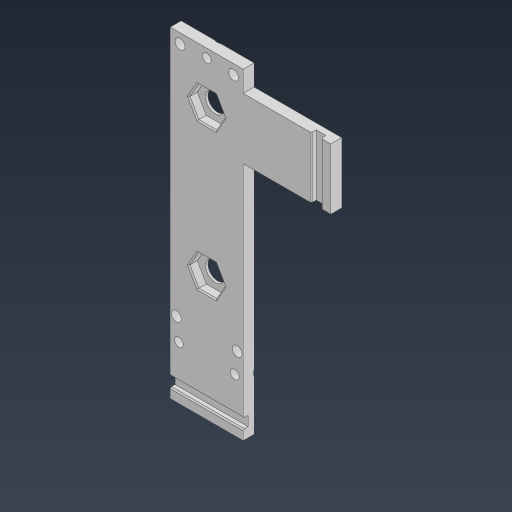
# Autodesk Inventor part: fusion_hold
Saved by Autodesk Inventor 2023 (Build 270158000, 158)
## iProperties
Created: 2025-12-26
Part Number: fusion_hold
Material: Generic
Document SubType Name: Modeling
Designer: szymo
Density: 1 g/cm^3
Appearance: Default
Author: szymo
Autodesk Inventor part; units mm, degrees
ref_plane "YZ Plane" through (0, 0, 0) normal (1, 0, 0) x (0, 1, 0)
ref_plane "XZ Plane" through (0, 0, 0) normal (0, 1, 0) x (-1, 0, 0)
ref_plane "XY Plane" through (0, 0, 0) normal (0, 0, 1) x (1, 0, 0)
ref_plane "Work Plane1" through (0, 0, 0) normal (0, 0, 1) x (1, 0, 0)
sketch "Sketch1" plane through (0, 0, 0) normal (0, 0, 1) x (1, 0, 0)
  line L0 (-10, -38.8003) -> (-10, -16.5003) projected
  arc A0 (-10, -38.8003) -> (-7.75, -41.0997) centre (-7.7, -38.8003) ccw projected
  arc A1 (-7.75, -41.0997) -> (-5.5, -38.8003) centre (-7.8, -38.8003) ccw projected
  line L1 (-5.5, -30.0003) -> (-5.5, -38.8003) projected
  arc A2 (5.5, -30.0003) -> (-5.5, -30.0003) centre (0, -30.0003) ccw projected
  line L2 (5.5, -38.8003) -> (5.5, -30.0003) projected
  arc A3 (5.5, -38.8003) -> (7.75, -41.0997) centre (7.8, -38.8003) ccw projected
  arc A4 (7.75, -41.0997) -> (10, -38.8003) centre (7.7, -38.8003) ccw projected
  line L3 (10, -16.5003) -> (10, -38.8003) projected
  line L4 (3.75, -16.5003) -> (10, -16.5003) projected
  line L5 (3.75, -12.5003) -> (3.75, -16.5003) projected
  line L6 (7.5, -12.5003) -> (3.75, -12.5003) projected
  line L7 (7.5, -10.0003) -> (7.5, -12.5003) projected
  line L8 (1.75, -10.0003) -> (7.5, -10.0003) projected
  arc A5 (1.25, -9.5003) -> (1.75, -10.0003) centre (1.75, -9.5003) ccw projected
  line L9 (1.25, 9.4997) -> (1.25, -9.5003) projected
  arc A6 (1.75, 9.9997) -> (1.25, 9.4997) centre (1.75, 9.4997) ccw projected
  line L10 (7.5, 9.9997) -> (1.75, 9.9997) projected
  line L11 (7.5, 12.4997) -> (7.5, 9.9997) projected
  line L12 (3.75, 12.4997) -> (7.5, 12.4997) projected
  line L13 (3.75, 16.4997) -> (3.75, 12.4997) projected
  line L14 (10, 16.4997) -> (3.75, 16.4997) projected
  line L15 (10, 21.6997) -> (10, 16.4997) projected
  arc A7 (10, 21.6997) -> (7.2, 24.4997) centre (7.2, 21.6997) ccw projected
  line L16 (0, 24.4997) -> (7.2, 24.4997) projected
  arc A8 (0, 35.4997) -> (0, 24.4997) centre (0, 29.9997) ccw projected
  line L17 (7.2, 35.4997) -> (0, 35.4997) projected
  arc A9 (7.2, 35.4997) -> (7.2, 41.0997) centre (7.2, 38.2997) ccw projected
  line L18 (-10, 41.0997) -> (7.2, 41.0997) projected
  line L19 (-10, 16.4997) -> (-10, 41.0997) projected
  line L20 (-3.75, 16.4997) -> (-10, 16.4997) projected
  line L21 (-3.75, 12.4997) -> (-3.75, 16.4997) projected
  line L22 (-7.5, 12.4997) -> (-3.75, 12.4997) projected
  line L23 (-7.5, 9.9997) -> (-7.5, 12.4997) projected
  line L24 (-1.75, 9.9997) -> (-7.5, 9.9997) projected
  arc A10 (-1.25, 9.4997) -> (-1.75, 9.9997) centre (-1.75, 9.4997) ccw projected
  line L25 (-1.25, -9.5003) -> (-1.25, 9.4997) projected
  arc A11 (-1.75, -10.0003) -> (-1.25, -9.5003) centre (-1.75, -9.5003) ccw projected
  line L26 (-7.5, -10.0003) -> (-1.75, -10.0003) projected
  line L27 (-7.5, -12.5003) -> (-7.5, -10.0003) projected
  line L28 (-3.75, -12.5003) -> (-7.5, -12.5003) projected
  line L29 (-3.75, -16.5003) -> (-3.75, -12.5003) projected
  line L30 (-10, -16.5003) -> (-3.75, -16.5003) projected
  line L31 (15, 51.0997) -> (-15, 51.0997)
  line L32 (-15, 51.0997) -> (-15, -81.0997)
  line L33 (-15, -81.0997) -> (15, -81.0997)
  line L34 (15, -81.0997) -> (15, 51.0997)
  circle A12 centre (0, 29.9997) radius 4
  circle A13 centre (0, -30.0003) radius 4
  line L35 (15, 18.4997) -> (-15, 18.4997)
  line L36 (-15, -18.5003) -> (15, -18.5003)
  line L37 (13.1, 18.4997) -> (13.1, -18.5003)
  line L38 (-13.1, -18.5003) -> (-13.1, 18.4997)
  line L39 (11.1, 15.3997) -> (11.1, -15.4003) projected
  line L40 (-11.1, 15.3997) -> (-11.1, -15.4003) projected
  point P0 (0, 0)
  point P1 (10, -18.5003)
  point P2 (-10, -18.5003)
  point P3 (-10, 18.4997)
  point P4 (10, 18.4997)
  dimension "d5" = 8
  dimension "d6" = 8
  dimension "d8" = 5
  dimension "d9" = 10
  dimension "d10" = 5
  dimension "d11" = 40
  dimension "d12" = 2
  dimension "d13" = 2
  dimension "d14" = 2
  dimension "d15" = 2
  constraints: 16 end point, 8 point on line, 5 parallel, 5 perpendicular, 2 centre point, 2 coincident, 1 horizontal
  measures "d5" diameter of A12
  measures "d6" diameter of A13
  measures "d8" distance between parallel lines of L19 L32
  measures "d9" distance between parallel lines of L31 L18
  measures "d10" distance between parallel lines of L34 L15
  measures "d11" distance from line of L33 A0.end
  measures "d12" distance between parallel lines of L20 L35
  measures "d13" distance between parallel lines of L36 L4
  measures "d14" distance between parallel lines of L39 L37
  measures "d15" distance between parallel lines of L40 L38
extrude "Extrusion1" add sketch "Sketch1" along normal blind 1 contours A0 A1 L1 A2 L2 A3 A4 L3 L36 L34 L33 L32 L0 | L0 L36 L3 A4 A3 L2 A2 L1 A1 A0 | L36 L32 L35 L38 | L35 L32 L31 L34 L15 A7 L16 A8 L17 A9 L18 L19 | L37 L35 L34 L36 | L19 L18 A9 L17 A8 L16 A7 L15 L35
sketch "Sketch2" plane through (0, 0, 1) normal (0, 0, 1) x (1, 0, 0)
  line L0 (15, 51.0997) -> (-15, 51.0997) projected
  line L1 (-15, 51.0997) -> (-15, -81.0997) projected
  line L2 (-15, -81.0997) -> (15, -81.0997) projected
  line L3 (15, -81.0997) -> (15, 51.0997) projected
  circle A0 centre (0, -30.0003) radius 4 projected
  line L4 (13.1, -18.5003) -> (-13.1, -18.5003) projected
  line L5 (-13.1, -18.5003) -> (-13.1, 18.4997) projected
  line L6 (-13.1, 18.4997) -> (13.1, 18.4997) projected
  line L7 (13.1, 18.4997) -> (13.1, -18.5003) projected
  circle A1 centre (0, 29.9997) radius 4 projected
  line L8 (3.695, 36.3997) -> (7.3901, 29.9997)
  line L9 (7.3901, 29.9997) -> (3.695, 23.5997)
  line L10 (3.695, 23.5997) -> (-3.695, 23.5997)
  line L11 (-3.695, 23.5997) -> (-7.3901, 29.9997)
  line L12 (-7.3901, 29.9997) -> (-3.695, 36.3997)
  line L13 (-3.695, 36.3997) -> (3.695, 36.3997)
  line L14 (7.3901, -30.0003) -> (3.695, -36.4003)
  line L15 (3.695, -36.4003) -> (-3.695, -36.4003)
  line L16 (-3.695, -36.4003) -> (-7.3901, -30.0003)
  line L17 (-7.3901, -30.0003) -> (-3.695, -23.6003)
  line L18 (-3.695, -23.6003) -> (3.695, -23.6003)
  line L19 (3.695, -23.6003) -> (7.3901, -30.0003)
  point P0 (0, 0)
  point P1 (0, 29.9997)
  point P2 (0, -30.0003)
  dimension "d20" = 0
  dimension "d21" = 0
  dimension "d22" = 12.8
  dimension "d23" = 12.8
  constraints: 24 end point, 2 coincident, 26 other
  measures "d20" angle of L2 L15
  measures "d21" angle of L0 L13
  measures "d22" distance between parallel lines of L10 L13
  measures "d23" distance between parallel lines of L15 L18
extrude "Extrusion2" add sketch "Sketch2" along normal blind 2 contours L3 L2 L1 L0
sketch "Sketch6" plane through (0, 0, 3) normal (0, 0, 1) x (1, 0, 0)
  line L0 (-15, 51.0997) -> (-15, -81.0997) projected
  line L1 (-15, -81.0997) -> (15, -81.0997) projected
  line L2 (15, -81.0997) -> (15, 51.0997) projected
  line L3 (15, 51.0997) -> (-15, 51.0997) projected
  line L4 (7.3901, -30.0003) -> (3.695, -36.4003) projected
  line L5 (3.695, -36.4003) -> (-3.695, -36.4003) projected
  line L6 (-3.695, -36.4003) -> (-7.3901, -30.0003) projected
  line L7 (-7.3901, -30.0003) -> (-3.695, -23.6003) projected
  line L8 (-3.695, -23.6003) -> (3.695, -23.6003) projected
  line L9 (3.695, -23.6003) -> (7.3901, -30.0003) projected
  line L10 (3.695, 36.3997) -> (7.3901, 29.9997) projected
  line L11 (7.3901, 29.9997) -> (3.695, 23.5997) projected
  line L12 (3.695, 23.5997) -> (-3.695, 23.5997) projected
  line L13 (-3.695, 23.5997) -> (-7.3901, 29.9997) projected
  line L14 (-7.3901, 29.9997) -> (-3.695, 36.3997) projected
  line L15 (-3.695, 36.3997) -> (3.695, 36.3997) projected
  line L16 (13.1, -18.5003) -> (-13.1, -18.5003) projected
  line L17 (-13.1, -18.5003) -> (-13.1, 18.4997) projected
  line L18 (-13.1, 18.4997) -> (13.1, 18.4997) projected
  line L19 (13.1, 18.4997) -> (13.1, -18.5003) projected
  point P0 (0, 0)
extrude "Extrusion3" add sketch "Sketch6" along normal blind 1.5 contours L3 L2 L1 L0 | L16 L17 L18 L19
sketch "Sketch7" plane through (0, 0, 0) normal (0, 0, -1) x (-1, 0, 0)
  line L0 (15, -81.0997) -> (-15, -81.0997) projected
  line L1 (0, -81.0997) -> (0, 51.0997)
  line L2 (-15, 51.0997) -> (15, 51.0997) projected
  circle A0 centre (0, 47.5997) radius 3.5
  line L3 (15, -81.0997) -> (-15, -81.0997) projected
  line L4 (10, -38.8003) -> (10, -16.5003) projected
  line L5 (10, -16.5003) -> (3.75, -16.5003) projected
  line L6 (3.75, -16.5003) -> (3.75, -12.5003) projected
  line L7 (3.75, -12.5003) -> (7.5, -12.5003) projected
  line L8 (7.5, -12.5003) -> (7.5, -10.0003) projected
  line L9 (7.5, -10.0003) -> (1.75, -10.0003) projected
  arc A1 (1.25, -9.5003) -> (1.75, -10.0003) centre (1.75, -9.5003) ccw projected
  line L10 (1.25, -9.5003) -> (1.25, 9.4997) projected
  arc A2 (1.75, 9.9997) -> (1.25, 9.4997) centre (1.75, 9.4997) ccw projected
  line L11 (1.75, 9.9997) -> (7.5, 9.9997) projected
  line L12 (7.5, 9.9997) -> (7.5, 12.4997) projected
  line L13 (7.5, 12.4997) -> (3.75, 12.4997) projected
  line L14 (3.75, 12.4997) -> (3.75, 16.4997) projected
  line L15 (3.75, 16.4997) -> (10, 16.4997) projected
  line L16 (10, 16.4997) -> (10, 41.0997) projected
  line L17 (10, 41.0997) -> (-7.2, 41.0997) projected
  arc A3 (-7.2, 41.0997) -> (-7.2, 35.4997) centre (-7.2, 38.2997) ccw projected
  line L18 (-7.2, 35.4997) -> (0, 35.4997) projected
  arc A4 (0, 24.4997) -> (0, 35.4997) centre (0, 29.9997) ccw projected
  line L19 (0, 24.4997) -> (-7.2, 24.4997) projected
  arc A5 (-7.2, 24.4997) -> (-10, 21.6997) centre (-7.2, 21.6997) ccw projected
  line L20 (-10, 21.6997) -> (-10, 16.4997) projected
  line L21 (-10, 16.4997) -> (-3.75, 16.4997) projected
  line L22 (-3.75, 16.4997) -> (-3.75, 12.4997) projected
  line L23 (-3.75, 12.4997) -> (-7.5, 12.4997) projected
  line L24 (-7.5, 12.4997) -> (-7.5, 9.9997) projected
  line L25 (-7.5, 9.9997) -> (-1.75, 9.9997) projected
  arc A6 (-1.25, 9.4997) -> (-1.75, 9.9997) centre (-1.75, 9.4997) ccw projected
  line L26 (-1.25, 9.4997) -> (-1.25, -9.5003) projected
  arc A7 (-1.75, -10.0003) -> (-1.25, -9.5003) centre (-1.75, -9.5003) ccw projected
  line L27 (-1.75, -10.0003) -> (-7.5, -10.0003) projected
  line L28 (-7.5, -10.0003) -> (-7.5, -12.5003) projected
  line L29 (-7.5, -12.5003) -> (-3.75, -12.5003) projected
  line L30 (-3.75, -12.5003) -> (-3.75, -16.5003) projected
  line L31 (-3.75, -16.5003) -> (-10, -16.5003) projected
  line L32 (-10, -16.5003) -> (-10, -38.8003) projected
  arc A8 (-10, -38.8003) -> (-7.75, -41.0997) centre (-7.7, -38.8003) ccw projected
  arc A9 (-7.75, -41.0997) -> (-5.5, -38.8003) centre (-7.8, -38.8003) ccw projected
  line L33 (-5.5, -38.8003) -> (-5.5, -30.0003) projected
  arc A10 (5.5, -30.0003) -> (-5.5, -30.0003) centre (0, -30.0003) ccw projected
  line L34 (5.5, -30.0003) -> (5.5, -38.8003) projected
  arc A11 (5.5, -38.8003) -> (7.75, -41.0997) centre (7.8, -38.8003) ccw projected
  arc A12 (7.75, -41.0997) -> (10, -38.8003) centre (7.7, -38.8003) ccw projected
  spline S0 degree 2 poles (8.3836, 27.626) (8.7269, 27.626) (9.1863, 27.1073) (9.1863, 26.7072) knots 0 0 0 1 2 2 2 projected
  spline S1 degree 2 poles (9.1863, 26.7072) (9.1863, 26.2922) (8.7516, 25.7908) (8.4107, 25.7908) knots 0 0 0 1 2 2 2 projected
  spline S2 degree 2 poles (8.4107, 25.7908) (8.2057, 25.7908) (7.8056, 26.0304) (7.692, 26.2552) knots 0 0 0 1 2 2 2 projected
  line L35 (7.692, 26.2552) -> (7.6796, 26.2552) projected
  spline S3 degree 2 poles (7.6796, 26.2552) (7.5561, 25.9884) (7.2004, 25.7142) (6.9188, 25.7142) knots 0 0 0 1 2 2 2 projected
  spline S4 degree 2 poles (6.9188, 25.7142) (6.5286, 25.7142) (6, 26.2823) (6, 26.7072) knots 0 0 0 1 2 2 2 projected
  spline S5 degree 2 poles (6, 26.7072) (6, 26.9344) (6.1359, 27.3074) (6.2618, 27.4383) knots 0 0 0 1 2 2 2 projected
  spline S6 degree 2 poles (6.2618, 27.4383) (6.3853, 27.5667) (6.7212, 27.7001) (6.9114, 27.7001) knots 0 0 0 1 2 2 2 projected
  spline S7 degree 2 poles (6.9114, 27.7001) (7.1584, 27.7001) (7.5734, 27.4358) (7.6969, 27.1839) knots 0 0 0 1 2 2 2 projected
  line L36 (7.6969, 27.1839) -> (7.7093, 27.1839) projected
  spline S8 degree 2 poles (7.7093, 27.1839) (7.8402, 27.4087) (8.1514, 27.626) (8.3836, 27.626) knots 0 0 0 1 2 2 2 projected
  spline S9 degree 2 poles (7.5932, 30.306) (6.7731, 30.306) (6.0049, 30.7827) (6.0049, 31.2792) knots 0 0 0 1 2 2 2 projected
  spline S10 degree 2 poles (6.0049, 31.2792) (6.0049, 31.7831) (6.7879, 32.2548) (7.5907, 32.2548) knots 0 0 0 1 2 2 2 projected
  spline S11 degree 2 poles (7.5907, 32.2548) (8.4157, 32.2548) (9.1789, 31.7781) (9.1789, 31.2792) knots 0 0 0 1 2 2 2 projected
  spline S12 degree 2 poles (9.1789, 31.2792) (9.1789, 30.7778) (8.3885, 30.306) (7.5932, 30.306) knots 0 0 0 1 2 2 2 projected
  spline S13 degree 2 poles (7.5907, 34.5421) (8.4157, 34.5421) (9.1789, 34.0653) (9.1789, 33.5664) knots 0 0 0 1 2 2 2 projected
  spline S14 degree 2 poles (9.1789, 33.5664) (9.1789, 33.065) (8.3885, 32.5932) (7.5932, 32.5932) knots 0 0 0 1 2 2 2 projected
  spline S15 degree 2 poles (7.5932, 32.5932) (6.7731, 32.5932) (6.0049, 33.0699) (6.0049, 33.5664) knots 0 0 0 1 2 2 2 projected
  spline S16 degree 2 poles (6.0049, 33.5664) (6.0049, 34.0703) (6.7879, 34.5421) (7.5907, 34.5421) knots 0 0 0 1 2 2 2 projected
  spline S17 degree 2 poles (7.0374, 28.0681) (6.8176, 28.0681) (6.4421, 28.2089) (6.3038, 28.3374) knots 0 0 0 1 2 2 2 projected
  spline S18 degree 2 poles (6.3038, 28.3374) (6.1655, 28.4658) (6.0049, 28.8487) (6.0049, 29.0858) knots 0 0 0 1 2 2 2 projected
  spline S19 degree 2 poles (6.0049, 29.0858) (6.0049, 29.3032) (6.1013, 29.728) (6.1778, 29.8836) knots 0 0 0 1 2 2 2 projected
  line L37 (6.1778, 29.8836) -> (6.6101, 29.8836) projected
  line L38 (6.6101, 29.8836) -> (6.6101, 29.854) projected
  spline S20 degree 2 poles (6.6101, 29.854) (6.5755, 29.807) (6.4866, 29.6317) (6.4471, 29.5255) knots 0 0 0 1 2 2 2 projected
  spline S21 degree 2 poles (6.4471, 29.5255) (6.4051, 29.4044) (6.3582, 29.2044) (6.3582, 29.0784) knots 0 0 0 1 2 2 2 projected
  spline S22 degree 2 poles (6.3582, 29.0784) (6.3582, 28.9549) (6.4471, 28.7227) (6.5434, 28.6387) knots 0 0 0 1 2 2 2 projected
  spline S23 degree 2 poles (6.5434, 28.6387) (6.6348, 28.5622) (6.8769, 28.4831) (7.0399, 28.4831) knots 0 0 0 1 2 2 2 projected
  spline S24 degree 2 poles (7.0399, 28.4831) (7.2029, 28.4831) (7.4104, 28.572) (7.4795, 28.656) knots 0 0 0 1 2 2 2 projected
  spline S25 degree 2 poles (7.4795, 28.656) (7.5561, 28.7425) (7.6203, 28.9993) (7.6203, 29.155) knots 0 0 0 1 2 2 2 projected
  spline S26 degree 2 poles (7.6203, 29.155) (7.6203, 29.3229) (7.5685, 29.6564) (7.5462, 29.7576) knots 0 0 0 1 2 2 2 projected
  line L39 (7.5462, 29.7576) -> (9.1172, 29.7576) projected
  line L40 (9.1172, 29.7576) -> (9.1172, 28.0854) projected
  line L41 (9.1172, 28.0854) -> (8.759, 28.0854) projected
  line L42 (8.759, 28.0854) -> (8.759, 29.3649) projected
  line L43 (8.759, 29.3649) -> (7.9464, 29.3649) projected
  spline S27 degree 2 poles (7.9464, 29.3649) (7.9563, 29.2908) (7.9637, 29.1475) (7.9637, 29.0883) knots 0 0 0 1 2 2 2 projected
  spline S28 degree 2 poles (7.9637, 29.0883) (7.9637, 28.8536) (7.8871, 28.53) (7.7735, 28.3818) knots 0 0 0 1 2 2 2 projected
  spline S29 degree 2 poles (7.7735, 28.3818) (7.6599, 28.2312) (7.314, 28.0681) (7.0374, 28.0681) knots 0 0 0 1 2 2 2 projected
  line L44 (6.0519, 36.5971) -> (6.4446, 36.5971) projected
  line L45 (6.4446, 36.5971) -> (6.4446, 36.5774) projected
  spline S30 degree 2 poles (6.4446, 36.5774) (6.415, 36.5255) (6.3631, 36.3081) (6.3631, 36.197) knots 0 0 0 1 2 2 2 projected
  spline S31 degree 2 poles (6.3631, 36.197) (6.3631, 35.7968) (6.8917, 35.3399) (7.3807, 35.3078) knots 0 0 0 1 2 2 2 projected
  spline S32 degree 2 poles (7.3807, 35.3078) (7.2696, 35.4708) (7.1683, 35.7672) (7.1683, 35.9426) knots 0 0 0 1 2 2 2 projected
  spline S33 degree 2 poles (7.1683, 35.9426) (7.1683, 36.1105) (7.2424, 36.3896) (7.3486, 36.5304) knots 0 0 0 1 2 2 2 projected
  spline S34 degree 2 poles (7.3486, 36.5304) (7.4746, 36.6934) (7.8575, 36.8614) (8.1267, 36.8614) knots 0 0 0 1 2 2 2 projected
  spline S35 degree 2 poles (8.1267, 36.8614) (8.3613, 36.8614) (8.7516, 36.7083) (8.8924, 36.5749) knots 0 0 0 1 2 2 2 projected
  spline S36 degree 2 poles (8.8924, 36.5749) (9.0282, 36.4489) (9.1789, 36.0809) (9.1789, 35.8932) knots 0 0 0 1 2 2 2 projected
  spline S37 degree 2 poles (9.1789, 35.8932) (9.1789, 35.6832) (9.0381, 35.3423) (8.9047, 35.2164) knots 0 0 0 1 2 2 2 projected
  spline S38 degree 2 poles (8.9047, 35.2164) (8.7368, 35.0583) (8.1934, 34.8854) (7.7759, 34.8854) knots 0 0 0 1 2 2 2 projected
  spline S39 degree 2 poles (7.7759, 34.8854) (7.398, 34.8854) (6.7212, 35.0558) (6.4965, 35.2213) knots 0 0 0 1 2 2 2 projected
  spline S40 degree 2 poles (6.4965, 35.2213) (6.2594, 35.3967) (6.0099, 35.8907) (6.0099, 36.2513) knots 0 0 0 1 2 2 2 projected
  spline S41 degree 2 poles (6.0099, 36.2513) (6.0099, 36.3328) (6.0272, 36.5181) (6.0519, 36.5971) knots 0 0 0 1 2 2 2 projected
  spline S42 degree 2 poles (7.5932, 23.4443) (6.7731, 23.4443) (6.0049, 23.921) (6.0049, 24.4175) knots 0 0 0 1 2 2 2 projected
  spline S43 degree 2 poles (6.0049, 24.4175) (6.0049, 24.9213) (6.7879, 25.3931) (7.5907, 25.3931) knots 0 0 0 1 2 2 2 projected
  spline S44 degree 2 poles (7.5907, 25.3931) (8.4157, 25.3931) (9.1789, 24.9164) (9.1789, 24.4175) knots 0 0 0 1 2 2 2 projected
  spline S45 degree 2 poles (9.1789, 24.4175) (9.1789, 23.9161) (8.3885, 23.4443) (7.5932, 23.4443) knots 0 0 0 1 2 2 2 projected
  circle A13 centre (-11.5, -59.2502) radius 3.5
  circle A14 centre (11.5, -59.2502) radius 3.5
  line L46 (15, 51.0997) -> (15, -81.0997) projected
  line L47 (-15, -81.0997) -> (-15, 51.0997) projected
  point P0 (0, 0)
  point P1 (0, -56.0997)
  dimension "d29" = 7
  dimension "d48" = 7
  dimension "d49" = 7
  dimension "d50" = 15
  dimension "d51" = 15
  constraints: 3 centre point, 3 tangent, 2 end point, 2 midpoint, 2 point on line
  measures "d29" diameter of A0
  measures "d48" diameter of A13
  measures "d49" diameter of A14
hole "Hole1" at (0, 47.5997, 0) at (11.5, -59.2502, 0) at (-11.5, -59.2502, 0) direction (0, 0, 1) diameter 3.6 depth 8.8 countersink diameter 7.5 countersink angle 90 clearance for "Countersunk Flat Head Screw ISO 2009/7046" size "M3" standard "ISO"
chamfer "Chamfer1" distance 0.5 angle 45 12 edges at (5.5426, -26.8003, 4.5) (5.5426, -33.2003, 4.5) (0, -36.4003, 4.5) (-5.5426, -33.2003, 4.5) (-5.5426, -26.8003, 4.5) (0, -23.6003, 4.5) (5.5426, 26.7997, 4.5) (5.5426, 33.1997, 4.5) (0, 36.3997, 4.5) (-5.5426, 33.1997, 4.5) (-5.5426, 26.7997, 4.5) (0, 23.5997, 4.5)
sketch "Sketch8" plane through (0, 0, 0) normal (0, 0, -1) x (-1, 0, 0)
  circle A0 centre (0, 29.9997) radius 4 projected
  line L0 (-13.1, -18.5003) -> (13.1, -18.5003) projected
  line L1 (-13.1, 18.4997) -> (-13.1, -18.5003) projected
  line L2 (13.1, 18.4997) -> (-13.1, 18.4997) projected
  line L3 (13.1, -18.5003) -> (13.1, 18.4997) projected
  circle A1 centre (0, -30.0003) radius 4 projected
  line L4 (-15, 51.0997) -> (-1.3463, 51.0997) projected
  line L5 (-15, -81.0997) -> (-15, -60.5965) projected
  line L6 (15, -81.0997) -> (-15, -81.0997) projected
  line L7 (15, 51.0997) -> (15, -57.9039) projected
  line L8 (10, -38.8003) -> (10, -16.5003) projected
  line L9 (10, -16.5003) -> (3.75, -16.5003) projected
  line L10 (3.75, -16.5003) -> (3.75, -12.5003) projected
  line L11 (3.75, -12.5003) -> (7.5, -12.5003) projected
  line L12 (7.5, -12.5003) -> (7.5, -10.0003) projected
  line L13 (7.5, -10.0003) -> (1.75, -10.0003) projected
  arc A2 (1.25, -9.5003) -> (1.75, -10.0003) centre (1.75, -9.5003) ccw projected
  line L14 (1.25, -9.5003) -> (1.25, 9.4997) projected
  arc A3 (1.75, 9.9997) -> (1.25, 9.4997) centre (1.75, 9.4997) ccw projected
  line L15 (1.75, 9.9997) -> (7.5, 9.9997) projected
  line L16 (7.5, 9.9997) -> (7.5, 12.4997) projected
  line L17 (7.5, 12.4997) -> (3.75, 12.4997) projected
  line L18 (3.75, 12.4997) -> (3.75, 16.4997) projected
  line L19 (3.75, 16.4997) -> (10, 16.4997) projected
  line L20 (10, 16.4997) -> (10, 41.0997) projected
  line L21 (10, 41.0997) -> (-7.2, 41.0997) projected
  arc A4 (-7.2, 41.0997) -> (-7.2, 35.4997) centre (-7.2, 38.2997) ccw projected
  line L22 (-7.2, 35.4997) -> (0, 35.4997) projected
  arc A5 (0, 24.4997) -> (0, 35.4997) centre (0, 29.9997) ccw projected
  line L23 (0, 24.4997) -> (-7.2, 24.4997) projected
  arc A6 (-7.2, 24.4997) -> (-10, 21.6997) centre (-7.2, 21.6997) ccw projected
  line L24 (-10, 21.6997) -> (-10, 16.4997) projected
  line L25 (-10, 16.4997) -> (-3.75, 16.4997) projected
  line L26 (-3.75, 16.4997) -> (-3.75, 12.4997) projected
  line L27 (-3.75, 12.4997) -> (-7.5, 12.4997) projected
  line L28 (-7.5, 12.4997) -> (-7.5, 9.9997) projected
  line L29 (-7.5, 9.9997) -> (-1.75, 9.9997) projected
  arc A7 (-1.25, 9.4997) -> (-1.75, 9.9997) centre (-1.75, 9.4997) ccw projected
  line L30 (-1.25, 9.4997) -> (-1.25, -9.5003) projected
  arc A8 (-1.75, -10.0003) -> (-1.25, -9.5003) centre (-1.75, -9.5003) ccw projected
  line L31 (-1.75, -10.0003) -> (-7.5, -10.0003) projected
  line L32 (-7.5, -10.0003) -> (-7.5, -12.5003) projected
  line L33 (-7.5, -12.5003) -> (-3.75, -12.5003) projected
  line L34 (-3.75, -12.5003) -> (-3.75, -16.5003) projected
  line L35 (-3.75, -16.5003) -> (-10, -16.5003) projected
  line L36 (-10, -16.5003) -> (-10, -38.8003) projected
  arc A9 (-10, -38.8003) -> (-7.75, -41.0997) centre (-7.7, -38.8003) ccw projected
  arc A10 (-7.75, -41.0997) -> (-5.5, -38.8003) centre (-7.8, -38.8003) ccw projected
  line L37 (-5.5, -38.8003) -> (-5.5, -30.0003) projected
  arc A11 (5.5, -30.0003) -> (-5.5, -30.0003) centre (0, -30.0003) ccw projected
  line L38 (5.5, -30.0003) -> (5.5, -38.8003) projected
  arc A12 (5.5, -38.8003) -> (7.75, -41.0997) centre (7.8, -38.8003) ccw projected
  arc A13 (7.75, -41.0997) -> (10, -38.8003) centre (7.7, -38.8003) ccw projected
  spline S0 degree 2 poles (8.3836, 27.626) (8.7269, 27.626) (9.1863, 27.1073) (9.1863, 26.7072) knots 0 0 0 1 2 2 2 projected
  spline S1 degree 2 poles (9.1863, 26.7072) (9.1863, 26.2922) (8.7516, 25.7908) (8.4107, 25.7908) knots 0 0 0 1 2 2 2 projected
  spline S2 degree 2 poles (8.4107, 25.7908) (8.2057, 25.7908) (7.8056, 26.0304) (7.692, 26.2552) knots 0 0 0 1 2 2 2 projected
  line L39 (7.692, 26.2552) -> (7.6796, 26.2552) projected
  spline S3 degree 2 poles (7.6796, 26.2552) (7.5561, 25.9884) (7.2004, 25.7142) (6.9188, 25.7142) knots 0 0 0 1 2 2 2 projected
  spline S4 degree 2 poles (6.9188, 25.7142) (6.5286, 25.7142) (6, 26.2823) (6, 26.7072) knots 0 0 0 1 2 2 2 projected
  spline S5 degree 2 poles (6, 26.7072) (6, 26.9344) (6.1359, 27.3074) (6.2618, 27.4383) knots 0 0 0 1 2 2 2 projected
  spline S6 degree 2 poles (6.2618, 27.4383) (6.3853, 27.5667) (6.7212, 27.7001) (6.9114, 27.7001) knots 0 0 0 1 2 2 2 projected
  spline S7 degree 2 poles (6.9114, 27.7001) (7.1584, 27.7001) (7.5734, 27.4358) (7.6969, 27.1839) knots 0 0 0 1 2 2 2 projected
  line L40 (7.6969, 27.1839) -> (7.7093, 27.1839) projected
  spline S8 degree 2 poles (7.7093, 27.1839) (7.8402, 27.4087) (8.1514, 27.626) (8.3836, 27.626) knots 0 0 0 1 2 2 2 projected
  spline S9 degree 2 poles (7.5932, 30.306) (6.7731, 30.306) (6.0049, 30.7827) (6.0049, 31.2792) knots 0 0 0 1 2 2 2 projected
  spline S10 degree 2 poles (6.0049, 31.2792) (6.0049, 31.7831) (6.7879, 32.2548) (7.5907, 32.2548) knots 0 0 0 1 2 2 2 projected
  spline S11 degree 2 poles (7.5907, 32.2548) (8.4157, 32.2548) (9.1789, 31.7781) (9.1789, 31.2792) knots 0 0 0 1 2 2 2 projected
  spline S12 degree 2 poles (9.1789, 31.2792) (9.1789, 30.7778) (8.3885, 30.306) (7.5932, 30.306) knots 0 0 0 1 2 2 2 projected
  spline S13 degree 2 poles (7.5907, 34.5421) (8.4157, 34.5421) (9.1789, 34.0653) (9.1789, 33.5664) knots 0 0 0 1 2 2 2 projected
  spline S14 degree 2 poles (9.1789, 33.5664) (9.1789, 33.065) (8.3885, 32.5932) (7.5932, 32.5932) knots 0 0 0 1 2 2 2 projected
  spline S15 degree 2 poles (7.5932, 32.5932) (6.7731, 32.5932) (6.0049, 33.0699) (6.0049, 33.5664) knots 0 0 0 1 2 2 2 projected
  spline S16 degree 2 poles (6.0049, 33.5664) (6.0049, 34.0703) (6.7879, 34.5421) (7.5907, 34.5421) knots 0 0 0 1 2 2 2 projected
  spline S17 degree 2 poles (7.0374, 28.0681) (6.8176, 28.0681) (6.4421, 28.2089) (6.3038, 28.3374) knots 0 0 0 1 2 2 2 projected
  spline S18 degree 2 poles (6.3038, 28.3374) (6.1655, 28.4658) (6.0049, 28.8487) (6.0049, 29.0858) knots 0 0 0 1 2 2 2 projected
  spline S19 degree 2 poles (6.0049, 29.0858) (6.0049, 29.3032) (6.1013, 29.728) (6.1778, 29.8836) knots 0 0 0 1 2 2 2 projected
  line L41 (6.1778, 29.8836) -> (6.6101, 29.8836) projected
  line L42 (6.6101, 29.8836) -> (6.6101, 29.854) projected
  spline S20 degree 2 poles (6.6101, 29.854) (6.5755, 29.807) (6.4866, 29.6317) (6.4471, 29.5255) knots 0 0 0 1 2 2 2 projected
  spline S21 degree 2 poles (6.4471, 29.5255) (6.4051, 29.4044) (6.3582, 29.2044) (6.3582, 29.0784) knots 0 0 0 1 2 2 2 projected
  spline S22 degree 2 poles (6.3582, 29.0784) (6.3582, 28.9549) (6.4471, 28.7227) (6.5434, 28.6387) knots 0 0 0 1 2 2 2 projected
  spline S23 degree 2 poles (6.5434, 28.6387) (6.6348, 28.5622) (6.8769, 28.4831) (7.0399, 28.4831) knots 0 0 0 1 2 2 2 projected
  spline S24 degree 2 poles (7.0399, 28.4831) (7.2029, 28.4831) (7.4104, 28.572) (7.4795, 28.656) knots 0 0 0 1 2 2 2 projected
  spline S25 degree 2 poles (7.4795, 28.656) (7.5561, 28.7425) (7.6203, 28.9993) (7.6203, 29.155) knots 0 0 0 1 2 2 2 projected
  spline S26 degree 2 poles (7.6203, 29.155) (7.6203, 29.3229) (7.5685, 29.6564) (7.5462, 29.7576) knots 0 0 0 1 2 2 2 projected
  line L43 (7.5462, 29.7576) -> (9.1172, 29.7576) projected
  line L44 (9.1172, 29.7576) -> (9.1172, 28.0854) projected
  line L45 (9.1172, 28.0854) -> (8.759, 28.0854) projected
  line L46 (8.759, 28.0854) -> (8.759, 29.3649) projected
  line L47 (8.759, 29.3649) -> (7.9464, 29.3649) projected
  spline S27 degree 2 poles (7.9464, 29.3649) (7.9563, 29.2908) (7.9637, 29.1475) (7.9637, 29.0883) knots 0 0 0 1 2 2 2 projected
  spline S28 degree 2 poles (7.9637, 29.0883) (7.9637, 28.8536) (7.8871, 28.53) (7.7735, 28.3818) knots 0 0 0 1 2 2 2 projected
  spline S29 degree 2 poles (7.7735, 28.3818) (7.6599, 28.2312) (7.314, 28.0681) (7.0374, 28.0681) knots 0 0 0 1 2 2 2 projected
  line L48 (6.0519, 36.5971) -> (6.4446, 36.5971) projected
  line L49 (6.4446, 36.5971) -> (6.4446, 36.5774) projected
  spline S30 degree 2 poles (6.4446, 36.5774) (6.415, 36.5255) (6.3631, 36.3081) (6.3631, 36.197) knots 0 0 0 1 2 2 2 projected
  spline S31 degree 2 poles (6.3631, 36.197) (6.3631, 35.7968) (6.8917, 35.3399) (7.3807, 35.3078) knots 0 0 0 1 2 2 2 projected
  spline S32 degree 2 poles (7.3807, 35.3078) (7.2696, 35.4708) (7.1683, 35.7672) (7.1683, 35.9426) knots 0 0 0 1 2 2 2 projected
  spline S33 degree 2 poles (7.1683, 35.9426) (7.1683, 36.1105) (7.2424, 36.3896) (7.3486, 36.5304) knots 0 0 0 1 2 2 2 projected
  spline S34 degree 2 poles (7.3486, 36.5304) (7.4746, 36.6934) (7.8575, 36.8614) (8.1267, 36.8614) knots 0 0 0 1 2 2 2 projected
  spline S35 degree 2 poles (8.1267, 36.8614) (8.3613, 36.8614) (8.7516, 36.7083) (8.8924, 36.5749) knots 0 0 0 1 2 2 2 projected
  spline S36 degree 2 poles (8.8924, 36.5749) (9.0282, 36.4489) (9.1789, 36.0809) (9.1789, 35.8932) knots 0 0 0 1 2 2 2 projected
  spline S37 degree 2 poles (9.1789, 35.8932) (9.1789, 35.6832) (9.0381, 35.3423) (8.9047, 35.2164) knots 0 0 0 1 2 2 2 projected
  spline S38 degree 2 poles (8.9047, 35.2164) (8.7368, 35.0583) (8.1934, 34.8854) (7.7759, 34.8854) knots 0 0 0 1 2 2 2 projected
  spline S39 degree 2 poles (7.7759, 34.8854) (7.398, 34.8854) (6.7212, 35.0558) (6.4965, 35.2213) knots 0 0 0 1 2 2 2 projected
  spline S40 degree 2 poles (6.4965, 35.2213) (6.2594, 35.3967) (6.0099, 35.8907) (6.0099, 36.2513) knots 0 0 0 1 2 2 2 projected
  spline S41 degree 2 poles (6.0099, 36.2513) (6.0099, 36.3328) (6.0272, 36.5181) (6.0519, 36.5971) knots 0 0 0 1 2 2 2 projected
  spline S42 degree 2 poles (7.5932, 23.4443) (6.7731, 23.4443) (6.0049, 23.921) (6.0049, 24.4175) knots 0 0 0 1 2 2 2 projected
  spline S43 degree 2 poles (6.0049, 24.4175) (6.0049, 24.9213) (6.7879, 25.3931) (7.5907, 25.3931) knots 0 0 0 1 2 2 2 projected
  spline S44 degree 2 poles (7.5907, 25.3931) (8.4157, 25.3931) (9.1789, 24.9164) (9.1789, 24.4175) knots 0 0 0 1 2 2 2 projected
  spline S45 degree 2 poles (9.1789, 24.4175) (9.1789, 23.9161) (8.3885, 23.4443) (7.5932, 23.4443) knots 0 0 0 1 2 2 2 projected
  line L50 (-15, -81.0997) -> (-15, 51.0997) projected
  line L51 (-15, 42.4997) -> (-51, 42.4997)
  line L52 (-51, 42.4997) -> (-51, 17.4997)
  line L53 (-51, 17.4997) -> (-15, 17.4997)
  arc A14 (-15, -60.5965) -> (-15, -57.9039) centre (-11.5, -59.2502) ccw projected
  line L54 (15, -60.5965) -> (15, -81.0997) projected
  arc A15 (15, -57.9039) -> (15, -60.5965) centre (11.5, -59.2502) ccw projected
  line L55 (1.3463, 51.0997) -> (15, 51.0997) projected
  arc A16 (-1.3463, 51.0997) -> (1.3463, 51.0997) centre (0, 47.5997) ccw projected
  line L56 (-15, -57.9039) -> (-15, 51.0997) projected
  point P0 (0, 0)
  point P1 (-15, 16.4997)
  point P2 (-15, 41.0997)
  dimension "d40" = 36
  dimension "d43" = 25
  dimension "d82" = 12.5
  dimension "d83" = 12.5
  constraints: 6 end point, 3 perpendicular, 2 point on line
  measures "d40" distance of L52.end L53.end
  measures "d43" distance of L51.end L52.end
  measures "d82" distance from line of L51 A0.centre
  measures "d83" distance from line of L53 A0.centre
extrude "Extrusion4" add sketch "Sketch8" against normal up to surface (4.5 mm away) contours L50 L53 L52 L51
sketch "Sketch9" plane through (-15, -81.0997, 4.5) normal (-1, 0, 0) x (0, 0, 1)
  line L0 (-4.5, 20.5032) -> (-4.5, 0) projected
  line L1 (-4.5, 0) -> (0, 0) projected
  line L2 (0, 132.1995) -> (0, 0) projected
  line L3 (-4.5, 132.1995) -> (0, 132.1995) projected
  line L4 (0, 0) -> (0, 132.1995) projected
  line L5 (0, 4) -> (-2, 4)
  line L6 (-2, 4) -> (-2, 8)
  line L7 (-2, 8) -> (0, 8)
  line L8 (-4.5, 132.1995) -> (-4.5, 23.1958) projected
  point P0 (-4.5, 81.0997)
  point P1 (0, 98.5995)
  point P2 (0, 4)
  point P3 (0, 8)
  dimension "d52" = 4
  dimension "d53" = 4
  dimension "d54" = 2.5
  dimension "d55" = 2
  constraints: 6 end point, 2 perpendicular, 2 point on line, 1 horizontal, 1 vertical alignment
  measures "d52" distance between parallel lines of L1 L5
  measures "d53" distance of L5.end L6.end
  measures "d54" distance between parallel lines of L0 L6
  measures "d55" distance between parallel lines of L2 L6
extrude "Extrusion5" cut sketch "Sketch9" against normal through all
sketch "Sketch10" plane through (15, 17.4997, 0) normal (0, -1, 0) x (1, 0, 0)
  line L0 (36, 4.5) -> (0, 4.5) projected
  line L1 (32, 4.5) -> (32, 2.5)
  line L2 (32, 2.5) -> (28, 2.5)
  line L3 (28, 2.5) -> (28, 4.5)
  line L4 (36, 0) -> (36, 4.5) projected
  point P0 (-15, 0)
  dimension "d61" = 4
  dimension "d62" = 4
  dimension "d63" = 2
  constraints: 6 end point, 3 perpendicular, 2 point on line
  measures "d61" distance between parallel lines of L4 L1
  measures "d62" distance of L1.end L2.end
  measures "d63" distance of L2.end L3.end
extrude "Extrusion6" cut sketch "Sketch10" against normal through all
chamfer "Chamfer2" distance 0.5 angle 45 4 edges at (0, -77.0997, 4.5) (0, -73.0997, 4.5) (43, 29.9997, 4.5) (47, 29.9997, 4.5)
sketch "Sketch11" plane through (0, 0, 0) normal (0, 0, -1) x (-1, 0, 0)
  line L0 (-15, -81.0997) -> (-15, 51.0997) projected
  line L1 (-15, -55.5002) -> (-10, -55.5002)
  line L2 (-10, -55.5002) -> (-10, -45.5002)
  line L3 (-10, -45.5002) -> (-15, -45.5002)
  line L4 (-15, -45.5002) -> (-15, -55.5002)
  arc A0 (-15, -60.5965) -> (-15, -57.9039) centre (-11.5, -59.2502) ccw projected
  line L5 (15, 51.0997) -> (15, -81.0997) projected
  line L6 (15, -55.5002) -> (10, -55.5002)
  line L7 (10, -55.5002) -> (10, -45.5002)
  line L8 (10, -45.5002) -> (15, -45.5002)
  line L9 (15, -45.5002) -> (15, -55.5002)
  arc A1 (15, -57.9039) -> (15, -60.5965) centre (11.5, -59.2502) ccw projected
  line L10 (-15, 51.0997) -> (15, 51.0997) projected
  line L11 (15, 51.0997) -> (7, 51.0997)
  line L12 (7, 51.0997) -> (7, 43.0997)
  line L13 (7, 43.0997) -> (15, 43.0997)
  line L14 (15, 43.0997) -> (15, 51.0997)
  line L15 (-15, 51.0997) -> (-7, 51.0997)
  line L16 (-7, 51.0997) -> (-7, 43.0997)
  line L17 (-7, 43.0997) -> (-15, 43.0997)
  line L18 (-15, 43.0997) -> (-15, 51.0997)
  line L19 (-15, -81.0997) -> (-15, 51.0997) projected
  line L20 (-15, -55.5002) -> (-10, -45.5002)
  line L21 (15, -45.5002) -> (10, -55.5002)
  line L22 (15, 51.0997) -> (7, 43.0997)
  line L23 (-15, 51.0997) -> (15, 51.0997) projected
  line L24 (-7, 43.0997) -> (-15, 51.0997)
  point P0 (0, 0)
  point P1 (-15, 17.4997)
  point P2 (1.3463, 51.0997)
  point P3 (-15, 42.4997)
  point P4 (-1.3463, 51.0997)
  point P5 (-12.5, -50.5002)
  point P6 (12.5, -50.5002)
  point P7 (11, 47.0997)
  point P8 (-11, 47.0997)
  dimension "d66" = 5
  dimension "d67" = 10
  dimension "d68" = 5
  dimension "d69" = 10
  dimension "d70" = 8
  dimension "d71" = 8
  dimension "d72" = 8
  dimension "d73" = 8
  constraints: 40 end point, 8 parallel, 4 horizontal, 4 midpoint, 4 perpendicular, 4 point on line, 2 tangent
  measures "d66" distance of L3.end L2.end
  measures "d67" distance of L2.end L1.end
  measures "d68" distance of L7.end L8.end
  measures "d69" distance of L6.end L7.end
  measures "d70" distance of L13.end L12.end
  measures "d71" distance of L12.end L11.end
  measures "d72" distance of L16.end L17.end
  measures "d73" distance of L15.end L16.end
hole "Hole2" at (12.5, -50.5002, 0) at (-12.5, -50.5002, 0) at (-11, 47.0997, 0) at (11, 47.0997, 0) direction (0, 0, 1) diameter 4 end through all counterbore diameter 4.5 counterbore depth 0.5
equation "\"d51\" = d50"
equation "\"d82\" = d83"
body "Solid1"
